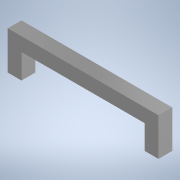
# Autodesk Inventor part: BarHandle5in
Saved by Autodesk Inventor 2022 (Build 260153000, 153)
## iProperties
Part Number: BarHandle5in
Material: Stainless Steel
Document SubType Name: Modeling
Designer: braxt
Density: 8 g/cm^3
Appearance: Semi-Polished
Author: braxt
Autodesk Inventor part; units mm, degrees
ref_plane "YZ Plane" through (0, 0, 0) normal (1, 0, 0) x (0, 1, 0)
ref_plane "XZ Plane" through (0, 0, 0) normal (0, 1, 0) x (-1, 0, 0)
ref_plane "XY Plane" through (0, 0, 0) normal (0, 0, 1) x (1, 0, 0)
sketch "Sketch1" plane through (0, 0, 0) normal (0, 0, 1) x (1, 0, 0)
  line L0 (0, 0) -> (12.7, 0)
  line L1 (12.7, 0) -> (12.7, 22.86)
  line L2 (0, 0) -> (0, 35.56)
  line L3 (0, 35.56) -> (139.7, 35.56)
  line L4 (139.7, 35.56) -> (139.7, 0.56)
  line L5 (139.7, 0.56) -> (127, 0.56)
  line L6 (127, 0.56) -> (127, 22.86)
  line L7 (127, 22.86) -> (12.7, 22.86)
  line L8 (6.35, 28.6931) -> (133.35, 28.6931) construction
  line L9 (6.35, 28.6931) -> (6.35, 0) construction
  line L10 (133.35, 28.6931) -> (133.35, 0) construction
  dimension "d0" = 12.7
  dimension "d2" = 35.56
  dimension "d4" = 12.7
  dimension "d28" = 12.7
  dimension "d29" = 127
  constraints: 22 end point, 6 perpendicular, 2 vertical, 1 horizontal, 1 midpoint, 1 parallel
  measures "d0" distance of L0.start L0.end
  measures "d2" distance of L0.start L2.end
  measures "d4" distance of L4.end L5.end
  measures "d28" distance between parallel lines of L3 L7
  measures "d29" distance of L8.start L8.end
extrude "Extrusion1" add sketch "Sketch1" along normal blind 12.7
hole "Hole1" at (6.35, 0, 6.35) direction (0, 1, 0) diameter 4.3434 depth 25 thread size "12-24 UNC" class "2B" standard "ANSI Unified Screw Threads"
hole "Hole2" at (133.35, 0.56, 6.35) direction (0, 1, 0) diameter 4.3434 depth 25 thread size "12-24 UNC" class "2B" standard "ANSI Unified Screw Threads"
body "Solid1"
